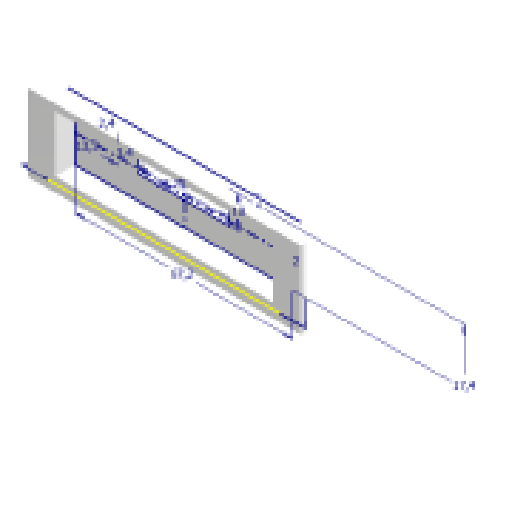
# Autodesk Inventor part: IR-housing
Saved by Autodesk Inventor 2026.1 (Build 301233020, 233B)
## iProperties
Created: 2026-02-21
Part Number: IR-housing
Material: ABS Plastic
Document SubType Name: Modeling
Designer: Snail
Density: 1.06 g/cm^3
Appearance: Smooth - White
Author: Snail
Autodesk Inventor part; units mm, degrees
ref_plane "YZ Plane" through (0, 0, 0) normal (1, 0, 0) x (0, 1, 0)
ref_plane "XZ Plane" through (0, 0, 0) normal (0, 1, 0) x (-1, 0, 0)
ref_plane "XY Plane" through (0, 0, 0) normal (0, 0, 1) x (1, 0, 0)
sketch "Sketch1" plane through (0, 0, 0) normal (0, 0, 1) x (1, 0, 0)
  line L0 (0, 0) -> (76, 0)
  line L1 (76, 0) -> (76, 17.4)
  line L2 (76, 17.4) -> (0, 17.4)
  line L3 (0, 17.4) -> (0, 0)
  line L4 (-2, 19.4) -> (78, 19.4)
  line L5 (78, 19.4) -> (78, -2)
  line L6 (78, -2) -> (-2, -2)
  line L7 (-2, -2) -> (-2, 19.4)
  line L8 (38, 0) -> (38, 17.4)
  line L9 (0, 8.7) -> (76, 8.7)
  line L10 (28, 17.4) -> (48, 17.4)
  line L11 (48, 17.4) -> (48, 7.4)
  line L12 (48, 7.4) -> (28, 7.4)
  line L13 (28, 7.4) -> (28, 17.4)
  line L14 (20, 15) -> (23.4, 15) construction
  line L15 (20, 12.6) -> (23.4, 12.6)
  line L16 (23.4, 17.4) -> (20, 17.4)
  arc A0 (20, 17.4) -> (20, 12.6) centre (20, 15) ccw
  arc A1 (23.4, 12.6) -> (23.4, 17.4) centre (23.4, 15) ccw
  line L17 (56, 12.6) -> (52.6, 12.6)
  line L18 (52.6, 17.4) -> (56, 17.4)
  arc A2 (56, 12.6) -> (56, 17.4) centre (56, 15) ccw
  arc A3 (52.6, 17.4) -> (52.6, 12.6) centre (52.6, 15) ccw
  point P0 (38, 7.4)
  point P1 (48, 17.4)
  point P2 (21.7, 15)
  dimension "d1" = 2
  dimension "d2" = 2
  dimension "d3" = 20
  dimension "d6" = 20
  dimension "d20" = 76
  dimension "d21" = 17.4
  dimension "d23" = 10
  dimension "d26" = 2.4
  dimension "d27" = 3.4
  constraints: 40 end point, 8 point on circle, 7 midpoint, 7 parallel, 6 symmetric about line, 4 centre point, 4 horizontal, 4 tangent, 3 perpendicular, 2 vertical alignment, 1 collinear, 1 point on line, 4 other
  measures "d1" distance between parallel lines of L4 L2
  measures "d2" distance between parallel lines of L5 L1
  measures "d3" distance from line of L3 L14.start
  measures "d6" distance of L11.end L12.end
  measures "d20" distance between parallel lines of L3 L1
  measures "d21" distance between parallel lines of L10 L0
  measures "d23" distance between parallel lines of L10 L12
  measures "d26" distance from line of L2 L14.start
  measures "d27" distance of L15.start L15.end
extrude "Extrusion1" add sketch "Sketch1" along normal blind 6.2
extrude "Extrusion2" add sketch "Sketch1" against normal blind 2 contours L3 L9 L13 L12 L8 L0 | L8 L12 L11 L9 L1 L0 | L3 L2 A0 L15 A1 L13 L9 | L9 L11 L2 A3 L17 A2 L1 | L2 A1 L15 A0 | A2 L17 A3 L2 | L4 L5 L6 L7
extrude "Extrusion3" cut sketch "Sketch1" against normal through all contours L2 A1 L15 A0 | A2 L17 A3 L2
sketch "Sketch2" plane through (-2, -2, 6.2) normal (0, -1, 0) x (1, 0, 0)
  line L0 (0, 0) -> (80, 0) projected
  line L1 (80, -8.2) -> (0, -8.2) projected
  line L2 (80, -8.2) -> (88.2, 0)
  line L3 (88.2, 0) -> (80, 0)
  line L4 (0, -8.2) -> (-8.2, 0)
  line L5 (-8.2, 0) -> (0, 0)
  line L6 (0.8284, -6.2) -> (79.1716, -6.2)
  line L7 (79.1716, -6.2) -> (83.3716, -2)
  line L8 (83.3716, -2) -> (71.2, -2)
  line L9 (71.2, -2) -> (0, -2)
  line L10 (0, -2) -> (-3.3716, -2)
  line L11 (-3.3716, -2) -> (0.8284, -6.2)
  line L12 (62.5973, -2) -> (57.9327, -6.2)
  line L13 (2, -6.2) -> (30, -6.2) projected
  line L14 (62.1752, -6.2) -> (66.3752, -2)
  line L15 (40, -8.2) -> (40, 0) construction
  line L16 (41.5, -6.2) -> (41.5, -2)
  line L17 (38.5, -6.2) -> (38.5, -2)
  line L18 (51.5944, -2) -> (47.3944, -6.2)
  line L19 (47.3518, -2) -> (43.1518, -6.2)
  line L20 (17.4027, -2) -> (22.0673, -6.2)
  line L21 (17.8248, -6.2) -> (13.6248, -2)
  line L22 (28.4056, -2) -> (32.6056, -6.2)
  line L23 (32.6482, -2) -> (36.8482, -6.2)
  point P0 (22.0673, -6.2)
  point P1 (17.4027, -2)
  point P2 (13.6248, -2)
  point P3 (17.8248, -6.2)
  point P4 (36.8482, -6.2)
  point P5 (32.6482, -2)
  point P6 (28.4056, -2)
  point P7 (32.6056, -6.2)
  dimension "d30" = 45
  dimension "d31" = 2
  dimension "d32" = 3
  dimension "d33" = 3
  dimension "d34" = 3
  constraints: 40 end point, 8 symmetric about line, 7 point on line, 3 collinear, 3 parallel, 2 midpoint, 2 perpendicular, 1 horizontal, 15 other
  measures "d30" angle of L3 L2
  measures "d32" distance between parallel lines of L17 L16
  measures "d33" angle of L14 L12
  measures "d34" distance between parallel lines of L19 L18
extrude "Extrusion4" add sketch "Sketch2" along normal blind 3
extrude "Extrusion5" add sketch "Sketch2" along normal blind 2 contours L21 L9 L20 L6 | L22 L9 L23 L6 | L17 L9 L16 L6 | L19 L9 L18 L6 | L12 L9 L14 L6
sketch "Sketch3" plane through (-2, -2, 6.2) normal (0, 1, 0) x (1, 0, 0)
  line L0 (80, 8.2) -> (80, 5.3716) projected
  line L1 (80, 2) -> (80, 0) projected
  line L2 (88.2, 0) -> (80, 0) projected
  line L3 (80, 8.2) -> (88.2, 0) projected
  line L4 (80, 8.2) -> (80, 5.3716) projected
  line L5 (83.3716, 2) -> (80, 5.3716) projected
  line L6 (80, 2) -> (83.3716, 2) projected
  line L7 (80, 2) -> (80, 0) projected
  line L8 (88.2, 0) -> (80, 0) projected
  line L9 (80, 8.2) -> (88.2, 0) projected
  line L10 (0, 5.3716) -> (0, 8.2) projected
  line L11 (-8.2, 0) -> (0, 8.2) projected
  line L12 (0, 0) -> (-8.2, 0) projected
  line L13 (0, 0) -> (0, 2) projected
  line L14 (-3.3716, 2) -> (0, 2) projected
  line L15 (0, 5.3716) -> (-3.3716, 2) construction
  line L16 (80, 5.3716) -> (80, 2) projected
  line L17 (0, 2) -> (0, 5.3716) projected
  line L18 (0, 8.2) -> (0, 0)
  point P0 (2, 6.2)
  constraints: 2 end point, 1 collinear
extrude "Extrusion6" add sketch "Sketch3" along normal up to surface (21.4 mm away)
fillet "Fillet2" radius 1 4 edges at (82.1, -5, 2.1) (38, -5, -2) (38, -5, 6.2) (-6.1, -5, 2.1)
fillet "Fillet3" radius 1 10 edges at (62.2752, -4, 2.1) (58.265, -4, 2.1) (47.4944, -4, 2.1) (43.2518, -4, 2.1) (39.5, -4, 2.1) (36.5, -4, 2.1) (32.7482, -4, 2.1) (28.5056, -4, 2.1) (17.735, -4, 2.1) (13.7248, -4, 2.1)
fillet "Fillet4" radius 1 4 edges at (-9.4929, -4.7071, 5.9071) (-10.2, 7.7, 6.2) (85.4929, -4.7071, 5.9071) (86.2, 7.7, 6.2)
body "Solid1"
